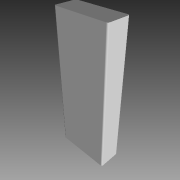
# Autodesk Inventor part: Casing_Generator
Saved by Autodesk Inventor 2016 (Build 200138000, 138)
## iProperties
Created: 2015-03-25
Part Number: Casing_Generator
Material: Générique
Document SubType Name: Modeling
Designer: Yann
Density: 1 g/cm^3
Appearance: Par défaut
Author: Yann
Autodesk Inventor part; units mm, degrees
ref_plane "YZ Plane" through (0, 0, 0) normal (1, 0, 0) x (0, 1, 0)
ref_plane "XZ Plane" through (0, 0, 0) normal (0, 1, 0) x (-1, 0, 0)
ref_plane "XY Plane" through (0, 0, 0) normal (0, 0, 1) x (1, 0, 0)
sketch "Esquisse1" plane through (0, 0, 0) normal (0, 1, 0) x (-1, 0, 0)
  line L0 (0, -308) -> (0, 308) construction
  line L1 (-119, 0) -> (119, 0) construction
  line L2 (-85, -220) -> (85, -220)
  line L3 (85, -220) -> (85, 220)
  line L4 (85, 220) -> (-85, 220)
  line L5 (-85, 220) -> (-85, -220)
  line L6 (-85, -220) -> (85, 220) construction
  line L7 (85, -220) -> (-85, 220) construction
  point P0 (0, 0)
  dimension "d0" = 170
  dimension "d1" = 440
  constraints: 12 end point, 2 midpoint, 2 parallel, 1 horizontal, 1 perpendicular
  measures "d0" distance of L4.end L3.end
  measures "d1" distance of L3.end L2.end
extrude "Extrusion1" add sketch "Esquisse1" along normal mid plane 70
fillet "Congé1" radius 5 4 edges at (85, -35, 0) (85, 35, 0) (-85, -35, 0) (-85, 35, 0)
